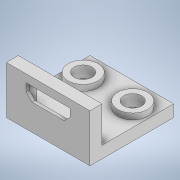
# Autodesk Inventor part: USBmicro
Saved by Autodesk Inventor 2022 (Build 260153000, 153)
## iProperties
Created: 2021-07-08
Part Number: USBmicro
Material: Generic
Document SubType Name: Modeling
Designer: anton
Density: 1 g/cm^3
Appearance: Default
Author: anton
Autodesk Inventor part; units mm, degrees
ref_plane "YZ Plane" through (0, 0, 0) normal (1, 0, 0) x (0, 1, 0)
ref_plane "XZ Plane" through (0, 0, 0) normal (0, 1, 0) x (-1, 0, 0)
ref_plane "XY Plane" through (0, 0, 0) normal (0, 0, 1) x (1, 0, 0)
sketch "Sketch1" plane through (0, 0, 0) normal (0, 1, 0) x (-1, 0, 0)
  line L0 (0, 0) -> (14, 0)
  line L1 (14, 0) -> (14, -14)
  line L2 (14, -14) -> (0, -14)
  line L3 (0, -14) -> (0, 0)
  dimension "d0" = 14
  dimension "d1" = 14
  constraints: 8 end point, 2 parallel, 1 horizontal, 1 perpendicular
  measures "d0" distance between parallel lines of L3 L1
  measures "d1" distance between parallel lines of L2 L0
extrude "Extrusion1" add sketch "Sketch1" along normal blind 2
sketch "Sketch2" plane through (0, 2, 0) normal (0, 1, 0) x (1, 0, 0)
  line L0 (-14, 14) -> (-14, 0) projected
  line L1 (0, 0) -> (-14, 0)
  line L2 (-14, 0) -> (-14, 2)
  line L3 (-14, 2) -> (0, 2)
  line L4 (0, 2) -> (0, 0)
  dimension "d4" = 2
  constraints: 8 end point, 2 parallel, 1 horizontal, 1 perpendicular, 1 point on line
  measures "d4" distance between parallel lines of L1 L3
extrude "Extrusion2" add sketch "Sketch2" along normal blind 6
sketch "Sketch3" plane through (0, 2, 0) normal (0, 1, 0) x (1, 0, 0)
  circle A0 centre (-11.15, 10) radius 2.5
  circle A1 centre (-2.85, 10) radius 2.5
  line L0 (-14, 0) -> (0, 0) projected
  line L1 (-14, 14) -> (-14, 2) projected
  line L2 (0, 2) -> (0, 14) projected
  dimension "d7" = 5
  dimension "d8" = 5
  dimension "d9" = 10
  dimension "d10" = 10
  dimension "d11" = 8.3
  dimension "d13" = 0.35
  constraints: 2 centre point
  measures "d7" diameter of A0
  measures "d8" diameter of A1
  measures "d9" distance from line of L0 A0.centre
  measures "d10" distance from line of L0 A1.centre
  measures "d11" distance of A1.centre A0.centre
  measures "d13" distance edge to line of A1 L2
extrude "Extrusion3" add sketch "Sketch3" along normal blind 1
sketch "Sketch4" plane through (-11.15, 3, -10) normal (0, 1, 0) x (1, 0, 0)
  circle A0 centre (8.3, 0) radius 2.5 projected
  circle A1 centre (8.3, 0) radius 1.5
  circle A2 centre (0, 0) radius 2.5 projected
  circle A3 centre (0, 0) radius 1.5
  point P0 (11.15, -10)
  dimension "d16" = 3
  dimension "d17" = 3
  constraints: 2 centre point, 2 coincident
  measures "d16" diameter of A3
  measures "d17" diameter of A1
extrude "Extrusion4" cut sketch "Sketch4" against normal blind 2 contours A1 | A3
sketch "Sketch5" plane through (0, 2, -2) normal (0, 0, -1) x (-1, 0, 0)
  line L0 (3.3, 4.7) -> (10.7, 4.7)
  line L1 (10.7, 4.7) -> (10.7, 3.4)
  line L2 (9.7, 2.4) -> (4.3, 2.4)
  line L3 (3.3, 3.4) -> (3.3, 4.7)
  line L4 (5.35, 1) -> (0.35, 1) projected
  line L5 (4.3, 2.4) -> (9.7, 2.4)
  line L6 (4.3, 2.4) -> (3.3, 3.4)
  line L7 (9.7, 2.4) -> (10.7, 3.4)
  line L8 (0, 0) -> (0, 6) projected
  point P0 (0, -2)
  dimension "d20" = 1.4
  dimension "d21" = 7.4
  dimension "d22" = 2.3
  dimension "d27" = 3.3
  dimension "d28" = 135
  dimension "d29" = 1
  dimension "d30" = 1
  constraints: 14 end point, 2 horizontal, 2 parallel, 2 perpendicular
  measures "d20" distance between parallel lines of L4 L2
  measures "d21" distance between parallel lines of L1 L3
  measures "d22" distance between parallel lines of L2 L0
  measures "d27" distance between parallel lines of L8 L3
  measures "d28" angle of L2 L6
  measures "d29" horizontal distance of L2.start L1.end
  measures "d30" horizontal distance of L2.end L3.start
extrude "Extrusion5" cut sketch "Sketch5" against normal blind 2
sketch "Sketch6" plane through (0, 2, -2) normal (0, 0, -1) x (-1, 0, 0)
  line L0 (14, 0) -> (0, 0) projected
  line L1 (3.1, 4.9) -> (10.9, 4.9)
  line L2 (10.9, 4.9) -> (10.9, 0)
  line L3 (10.9, 0) -> (3.1, 0)
  line L4 (3.1, 0) -> (3.1, 4.9)
  line L5 (3.3, 4.7) -> (10.7, 4.7) projected
  line L6 (3.3, 3.4) -> (3.3, 4.7) projected
  line L7 (10.7, 4.7) -> (10.7, 3.4) projected
  point P0 (0, -2)
  point P1 (3.1, 0)
  dimension "d33" = 0.2
  dimension "d34" = 0.2
  dimension "d35" = 0.2
  constraints: 8 end point, 2 parallel, 1 horizontal, 1 perpendicular, 1 point on line
  measures "d33" distance between parallel lines of L5 L1
  measures "d34" distance between parallel lines of L6 L4
  measures "d35" distance between parallel lines of L7 L2
extrude "Extrusion6" cut sketch "Sketch6" against normal blind 1.5
body "Solid1"
